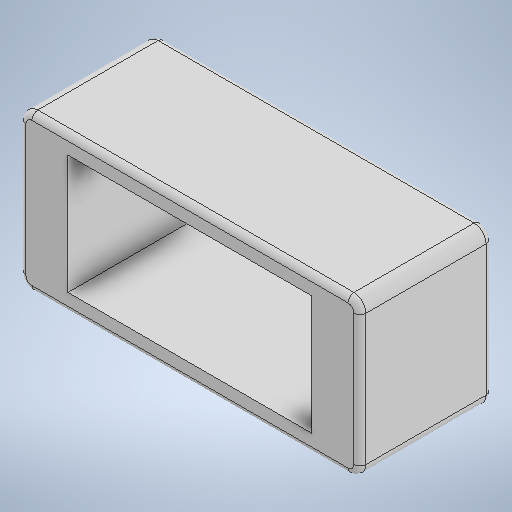
# Autodesk Inventor part: servo_to_links
Saved by Autodesk Inventor 2025 (Build 290162000, 162)
## iProperties
Created: 2024-05-25
Part Number: servo_to_links
Material: Generic
Document SubType Name: Modeling
Designer: hifzh
Density: 1 g/cm^3
Appearance: Default
Author: hifzh
Autodesk Inventor part; units mm, degrees
ref_plane "YZ Plane" through (0, 0, 0) normal (1, 0, 0) x (0, 1, 0)
ref_plane "XZ Plane" through (0, 0, 0) normal (0, 1, 0) x (-1, 0, 0)
ref_plane "XY Plane" through (0, 0, 0) normal (0, 0, 1) x (1, 0, 0)
sketch "Sketch1" plane through (0, 0, 0) normal (0, 0, 1) x (1, 0, 0)
  line L0 (0, 0) -> (0, 25.8)
  line L1 (0, 25.8) -> (56.6, 25.8)
  line L2 (56.6, 25.8) -> (56.6, 0)
  line L3 (56.6, 0) -> (0, 0)
  line L4 (8, 22.8) -> (48.6, 22.8)
  line L5 (48.6, 22.8) -> (48.6, 3)
  line L6 (48.6, 3) -> (8, 3)
  line L7 (8, 3) -> (8, 22.8)
  point P0 (28.3, 22.8)
  point P1 (28.3, 25.8)
  point P2 (28.3, 3)
  point P3 (56.6, 12.9)
  point P4 (48.6, 12.9)
  dimension "d0" = 56.6
  dimension "d1" = 25.8
  dimension "d2" = 40.6
  dimension "d3" = 19.8
  dimension "d4" = 3
  dimension "d5" = 3
  dimension "d6" = 8
  dimension "d7" = 8
  constraints: 16 end point, 6 perpendicular, 5 midpoint, 1 horizontal, 1 vertical
  measures "d0" distance of L0.end L1.end
  measures "d1" distance of L1.end L2.end
  measures "d2" distance of L4.start L4.end
  measures "d3" distance of L4.end L5.end
  measures "d4" distance of point (28.3, 22.8) point (28.3, 25.8)
  measures "d5" distance from line of L3 point (28.3, 3)
  measures "d6" distance between parallel lines of L0 L7
  measures "d7" distance of point (56.6, 12.9) point (48.6, 12.9)
extrude "Extrusion1" add sketch "Sketch1" along normal blind 22
fillet "Fillet1" radius 2 4 edges at (0, 0, 11) (0, 25.8, 11) (56.6, 25.8, 11) (56.6, 0, 11)
fillet "Fillet2" radius 1 16 edges at (0, 12.9, 22) (0.5858, 25.2142, 22) (28.3, 25.8, 22) (56.0142, 25.2142, 22) (56.6, 12.9, 22) (56.0142, 0.5858, 22) (28.3, 0, 22) (0.5858, 0.5858, 22) (28.3, 0, 0) (56.0142, 0.5858, 0) (56.6, 12.9, 0) (56.0142, 25.2142, 0) (28.3, 25.8, 0) (0.5858, 25.2142, 0) (0, 12.9, 0) (0.5858, 0.5858, 0)
body "Solid1"
